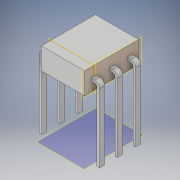
# Autodesk Inventor part: DetalV2(legs)
Saved by Autodesk Inventor 2018 (Build 220112000, 112)
## iProperties
Created: 2020-05-15
Part Number: DetalV2(legs)
Material: Generic
Document SubType Name: Modeling
Designer: User
Density: 1 g/cm^3
Appearance: Default
Author: User
Autodesk Inventor part; units mm, degrees
ref_plane "YZ Plane" through (0, 0, 0) normal (1, 0, 0) x (0, 1, 0)
ref_plane "XZ Plane" through (0, 0, 0) normal (0, 1, 0) x (-1, 0, 0)
ref_plane "XY Plane" through (0, 0, 0) normal (0, 0, 1) x (1, 0, 0)
sketch "Sketch2" plane through (0, 0, 0) normal (0, 0, 1) x (1, 0, 0)
  line L0 (3, -1.5) -> (-3, -1.5)
  line L1 (-3, -1.5) -> (-3, 1.5)
  line L2 (-3, 1.5) -> (3, 1.5)
  line L3 (3, 1.5) -> (3, -1.5)
  line L4 (3, -1.5) -> (-3, 1.5) construction
  line L5 (-3, -1.5) -> (3, 1.5) construction
  point P0 (0, 0)
  dimension "d4" = 6
  dimension "d5" = 3
  constraints: 12 end point, 2 midpoint, 2 parallel, 1 horizontal, 1 perpendicular
  measures "d4" distance of L1.end L2.end
  measures "d5" distance of L0.end L1.end
extrude "Extrusion1" add sketch "Sketch2" along normal mid plane 7.5
ref_plane "Work Plane1" through (3, -1.5, 3.75) normal (1, 0, 0) x (0, 0, -1)
ref_plane "Work Plane4" through (0, 0, 2.5) normal (0, 0, 1) x (1, 0, 0)
ref_plane "Work Plane5" through (-3, -10, 3.75) normal (0, -1, 0) x (1, 0, 0)
sketch "Sketch25" plane through (0, 0, 2.5) normal (0, 0, 1) x (1, 0, 0)
  line L0 (3, -1.5) -> (3, 1.5) projected
  line L1 (3, 0) -> (3.5, 0)
  line L2 (4, -0.5) -> (4, -10)
  arc A0 (4, -0.5) -> (3.5, 0) centre (3.5, -0.5) ccw
  point P0 (0, 0)
  point P1 (4, 0)
  dimension "d44" = 1
  dimension "d45" = 10
  dimension "d46" = 0.5
  constraints: 4 end point, 2 point on circle, 2 point on line, 2 tangent, 1 centre point, 1 horizontal, 1 midpoint, 1 perpendicular
  measures "d44" distance of L1.start point (4, 0)
  measures "d45" distance of point (4, 0) L2.end
  measures "d46" radius of A0
sketch "Sketch26" plane through (-3, -10, 3.75) normal (0, -1, 0) x (1, 0, 0)
  line L0 (6.824, -0.8954) -> (7.174, -0.8954)
  line L1 (7.174, -0.8954) -> (7.174, -1.5954)
  line L2 (7.174, -1.5954) -> (6.824, -1.5954)
  line L3 (6.824, -1.5954) -> (6.824, -0.8954)
  line L4 (6.824, -0.8954) -> (7.174, -1.5954) construction
  line L5 (7.174, -0.8954) -> (6.824, -1.5954) construction
  point P0 (3, -3.75)
  point P1 (6.999, -1.2454)
  dimension "d37" = 0.35
  dimension "d38" = 0.7
  constraints: 12 end point, 2 midpoint, 2 parallel, 1 horizontal, 1 perpendicular
  measures "d37" distance of L1.end L2.end
  measures "d38" distance of L0.end L1.end
sweep "Sweep2" add profiles "Sketch26" path "Sketch25" path curves L2 A0 L1
pattern_linear "Rectangular Pattern2" count 3 spacing 2.5 along (0, 0, -1) of "Sweep2"
mirror "Mirror2" about plane through (0, 0, 0) normal (1, 0, 0) of "Sweep2", "Rectangular Pattern2"
body "Solid1"
